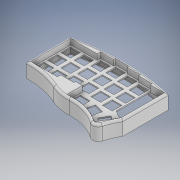
# Autodesk Inventor part: curvy
Saved by Autodesk Inventor 2021 (Build 250183000, 183)
## iProperties
Created: 2022-05-13
Part Number: curvy
Material: Generic
Document SubType Name: Modeling
Designer: Mark
Density: 1 g/cm^3
Appearance: Default
Author: Mark
Autodesk Inventor part; units mm, degrees
ref_plane "YZ Plane" through (0, 0, 0) normal (1, 0, 0) x (0, 1, 0)
ref_plane "XZ Plane" through (0, 0, 0) normal (0, 1, 0) x (-1, 0, 0)
ref_plane "XY Plane" through (0, 0, 0) normal (0, 0, 1) x (1, 0, 0)
sketch "keyholes" plane through (0, 0, 0) normal (0, 0, 1) x (1, 0, 0)
  line L0 (76.8681, -69.6062) -> (62.8681, -69.6062)
  line L1 (62.8681, -69.6062) -> (62.8681, -55.6062)
  line L2 (62.8681, -55.6062) -> (76.8681, -55.6062)
  line L3 (76.8681, -55.6062) -> (76.8681, -69.6062)
  line L4 (76.8681, -50.6062) -> (62.8681, -50.6062)
  line L5 (62.8681, -50.6062) -> (62.8681, -36.6062)
  line L6 (62.8681, -36.6062) -> (76.8681, -36.6062)
  line L7 (76.8681, -36.6062) -> (76.8681, -50.6062)
  line L8 (76.8681, -31.6062) -> (62.8681, -31.6062)
  line L9 (62.8681, -31.6062) -> (62.8681, -17.6062)
  line L10 (62.8681, -17.6062) -> (76.8681, -17.6062)
  line L11 (76.8681, -17.6062) -> (76.8681, -31.6062)
  point P0 (69.8681, -43.6062)
  dimension "d0" = 14
  dimension "d1" = 14
  dimension "d2" = 14
  dimension "d3" = 14
  dimension "d4" = 14
  dimension "d5" = 14
  dimension "d6" = 5
  dimension "d7" = 5
  measures "d0" distance of L1.end L2.end
  measures "d1" distance of L0.end L1.end
  measures "d2" distance of L5.end L6.end
  measures "d3" distance of L4.end L5.end
  measures "d4" distance of L9.end L10.end
  measures "d5" distance of L8.end L9.end
  measures "d6" distance between parallel lines of L4 L2
  measures "d7" distance between parallel lines of L8 L6
sketch "Sketch1" plane through (0, 0, 0) normal (0, 1, 0) x (-1, 0, 0)
  line L0 (119.155, -84.8943) -> (82.155, -84.8943) construction
  line L1 (64.1602, -28.6437) -> (119.155, -28.6437) construction
  line L2 (119.655, -29.1437) -> (119.655, -84.3943) construction
  line L3 (81.655, -85.3943) -> (81.655, -89.1443) construction
  line L4 (81.155, -89.6443) -> (63.155, -89.6443) construction
  line L5 (62.655, -90.1443) -> (62.655, -91.3943) construction
  line L6 (62.155, -91.8943) -> (45.155, -91.8943) construction
  line L7 (44.655, -91.3943) -> (44.655, -90.1443) construction
  line L8 (44.155, -89.6443) -> (26.155, -89.6443) construction
  line L9 (25.655, -89.1443) -> (25.655, -87.645) construction
  line L10 (25.155, -87.145) -> (7.155, -87.145) construction
  line L11 (63.7562, -28.4383) -> (53.3017, -14.1027) construction
  line L12 (52.9623, -13.9015) -> (15.7765, -9.0643) construction
  line L13 (15.591, -9.0015) -> (0.433, -0.25) construction
  line L14 (-0.25, -0.433) -> (-13.766, -23.8434) construction
  line L15 (-13.766, -23.8434) -> (6.655, -35.6335) construction
  line L16 (51.1256, -15.8625) -> (37.1256, -15.8625)
  line L17 (37.1256, -15.8625) -> (37.1256, -29.8625)
  line L18 (37.1256, -29.8625) -> (51.1256, -29.8625)
  line L19 (51.1256, -29.8625) -> (51.1256, -15.8625)
  line L20 (28.1127, -28.7255) -> (14.5898, -25.1021)
  line L21 (14.5898, -25.1021) -> (18.2132, -11.5791)
  line L22 (18.2132, -11.5791) -> (31.7362, -15.2026)
  line L23 (31.7362, -15.2026) -> (28.1127, -28.7255)
  line L24 (6.155, -84.895) -> (-13.5994, -84.895) construction
  line L25 (-14.0994, -84.395) -> (-14.0994, -24.5548) construction
  line L26 (-13.766, -23.8434) -> (-14.0324, -24.3048) construction
  line L27 (-8.6572, -18.9744) -> (-1.6572, -6.85)
  line L28 (3.4672, -25.9744) -> (-8.6572, -18.9744)
  line L29 (-1.6572, -6.85) -> (10.4672, -13.85)
  line L30 (10.4672, -13.85) -> (3.4672, -25.9744)
  arc A0 (119.155, -84.8943) -> (119.655, -84.3943) centre (119.155, -84.3943) ccw construction
  arc A1 (82.155, -84.8943) -> (81.655, -85.3943) centre (82.155, -85.3943) ccw construction
  arc A2 (81.155, -89.6443) -> (81.655, -89.1443) centre (81.155, -89.1443) ccw construction
  arc A3 (62.155, -91.8943) -> (62.655, -91.3943) centre (62.155, -91.3943) ccw construction
  arc A4 (44.655, -90.1443) -> (44.155, -89.6443) centre (44.155, -90.1443) ccw construction
  arc A5 (44.655, -91.3943) -> (45.155, -91.8943) centre (45.155, -91.3943) ccw construction
  arc A6 (63.155, -89.6443) -> (62.655, -90.1443) centre (63.155, -90.1443) ccw construction
  arc A7 (25.655, -89.1443) -> (26.155, -89.6443) centre (26.155, -89.1443) ccw construction
  arc A8 (-14.0994, -84.395) -> (-13.5994, -84.895) centre (-13.5994, -84.395) ccw construction
  line L31 (6.655, -86.645) -> (6.655, -85.395) construction
  arc A9 (25.655, -87.645) -> (25.155, -87.145) centre (25.155, -87.645) ccw construction
  arc A10 (6.655, -86.645) -> (7.155, -87.145) centre (7.155, -86.645) ccw construction
  arc A11 (6.655, -85.395) -> (6.155, -84.895) centre (6.155, -85.395) ccw construction
  arc A12 (-14.0324, -24.3048) -> (-14.0994, -24.5548) centre (-13.5994, -24.5548) ccw construction
  arc A13 (0.433, -0.25) -> (-0.25, -0.433) centre (0.183, -0.683) ccw construction
  arc A14 (15.591, -9.0015) -> (15.7765, -9.0643) centre (15.841, -8.5685) ccw construction
  arc A15 (53.3017, -14.1027) -> (52.9623, -13.9015) centre (52.8978, -14.3973) ccw construction
  arc A16 (63.7562, -28.4383) -> (64.1602, -28.6437) centre (64.1602, -28.1437) ccw construction
  arc A17 (119.655, -29.1437) -> (119.155, -28.6437) centre (119.155, -29.1437) ccw construction
  line L32 (6.655, -35.6335) -> (6.655, -85.395) construction
  line L33 (120.144, -28.2713) -> (120.144, -85.2713)
  line L34 (120.144, -85.2713) -> (82.144, -85.2713)
  line L35 (82.144, -85.2713) -> (82.144, -90.0161)
  line L36 (82.144, -90.0161) -> (63.144, -90.0161)
  line L37 (63.144, -90.0161) -> (63.144, -92.395)
  line L38 (63.144, -92.395) -> (44.144, -92.395)
  line L39 (44.144, -92.395) -> (44.144, -90.0204)
  line L40 (44.144, -90.0204) -> (25.144, -90.0204)
  line L41 (25.144, -90.0204) -> (25.144, -87.6356)
  line L42 (25.144, -87.6356) -> (6.144, -87.6356)
  line L43 (120.144, -28.2713) -> (82.144, -28.2713)
  line L44 (82.144, -28.2713) -> (82.144, -33.0161)
  line L45 (82.144, -33.0161) -> (63.144, -33.0161)
  line L46 (63.144, -33.0161) -> (63.144, -35.395)
  line L47 (63.144, -35.395) -> (53.6256, -35.395)
  line L48 (53.6256, -35.395) -> (53.6256, -13.3625)
  line L49 (53.6256, -13.3625) -> (34.5282, -13.3625)
  line L50 (34.5282, -13.3625) -> (16.0445, -8.4098)
  line L51 (16.0445, -8.4098) -> (-0.0722, 0.8952)
  line L52 (-0.0722, 0.8952) -> (-14.5722, -24.2195)
  line L53 (-14.5722, -24.2195) -> (6.144, -36.1801)
  line L54 (6.144, -36.1801) -> (6.144, -87.6356)
  line L55 (6.155, -84.895) -> (-14.0994, -84.895)
  arc A18 (73.017, -18.1715) -> (120.144, -28.2713) centre (120.144, 86.7287) ccw
  arc A19 (-14.0994, -84.895) -> (120.144, -85.2713) centre (53.8578, 212.9425) ccw
  arc A20 (-0.0722, 0.8952) -> (53.6256, -13.3625) centre (44.1644, 59.2526) ccw construction
  arc A21 (2.09, 0.0448) -> (47.4821, -13.3064) centre (44.1644, 59.2526) ccw
  arc A22 (-14.0994, -23.4005) -> (-5.3538, -2.5918) centre (-92.0416, 21.5995) ccw
  line L56 (-14.0994, -84.895) -> (-14.0994, -23.4005)
  arc A23 (73.017, -18.1715) -> (47.4821, -13.3064) centre (50.0429, -69.3097) ccw
  arc A24 (2.09, 0.0448) -> (-5.3538, -2.5918) centre (-0.7055, -3.889) ccw
  line L57 (98.644, -82.7713) -> (84.644, -82.7713)
  line L58 (84.644, -82.7713) -> (84.644, -68.7713)
  line L59 (84.644, -68.7713) -> (98.644, -68.7713)
  line L60 (98.644, -68.7713) -> (98.644, -82.7713)
  line L61 (98.644, -63.7713) -> (84.644, -63.7713)
  line L62 (84.644, -63.7713) -> (84.644, -49.7713)
  line L63 (84.644, -49.7713) -> (98.644, -49.7713)
  line L64 (98.644, -49.7713) -> (98.644, -63.7713)
  line L65 (98.644, -44.7713) -> (84.644, -44.7713)
  line L66 (84.644, -44.7713) -> (84.644, -30.7713)
  line L67 (84.644, -30.7713) -> (98.644, -30.7713)
  line L68 (98.644, -30.7713) -> (98.644, -44.7713)
  line L69 (117.644, -82.7713) -> (103.644, -82.7713)
  line L70 (103.644, -82.7713) -> (103.644, -68.7713)
  line L71 (103.644, -68.7713) -> (117.644, -68.7713)
  line L72 (117.644, -68.7713) -> (117.644, -82.7713)
  line L73 (117.644, -63.7713) -> (103.644, -63.7713)
  line L74 (103.644, -63.7713) -> (103.644, -49.7713)
  line L75 (103.644, -49.7713) -> (117.644, -49.7713)
  line L76 (117.644, -49.7713) -> (117.644, -63.7713)
  line L77 (117.644, -44.7713) -> (103.644, -44.7713)
  line L78 (103.644, -44.7713) -> (103.644, -30.7713)
  line L79 (103.644, -30.7713) -> (117.644, -30.7713)
  line L80 (117.644, -30.7713) -> (117.644, -44.7713)
  line L81 (79.644, -87.5161) -> (65.644, -87.5161)
  line L82 (65.644, -87.5161) -> (65.644, -73.5161)
  line L83 (65.644, -73.5161) -> (79.644, -73.5161)
  line L84 (79.644, -73.5161) -> (79.644, -87.5161)
  line L85 (79.644, -68.5161) -> (65.644, -68.5161)
  line L86 (65.644, -68.5161) -> (65.644, -54.5161)
  line L87 (65.644, -54.5161) -> (79.644, -54.5161)
  line L88 (79.644, -54.5161) -> (79.644, -68.5161)
  line L89 (79.644, -49.5161) -> (65.644, -49.5161)
  line L90 (65.644, -49.5161) -> (65.644, -35.5161)
  line L91 (65.644, -35.5161) -> (79.644, -35.5161)
  line L92 (79.644, -35.5161) -> (79.644, -49.5161)
  line L93 (60.644, -89.895) -> (46.644, -89.895)
  line L94 (46.644, -89.895) -> (46.644, -75.895)
  line L95 (46.644, -75.895) -> (60.644, -75.895)
  line L96 (60.644, -75.895) -> (60.644, -89.895)
  line L97 (60.644, -70.895) -> (46.644, -70.895)
  line L98 (46.644, -70.895) -> (46.644, -56.895)
  line L99 (46.644, -56.895) -> (60.644, -56.895)
  line L100 (60.644, -56.895) -> (60.644, -70.895)
  line L101 (60.644, -51.895) -> (46.644, -51.895)
  line L102 (46.644, -51.895) -> (46.644, -37.895)
  line L103 (46.644, -37.895) -> (60.644, -37.895)
  line L104 (60.644, -37.895) -> (60.644, -51.895)
  line L105 (41.644, -87.5204) -> (27.644, -87.5204)
  line L106 (27.644, -87.5204) -> (27.644, -73.5204)
  line L107 (27.644, -73.5204) -> (41.644, -73.5204)
  line L108 (41.644, -73.5204) -> (41.644, -87.5204)
  line L109 (41.644, -68.5204) -> (27.644, -68.5204)
  line L110 (27.644, -68.5204) -> (27.644, -54.5204)
  line L111 (27.644, -54.5204) -> (41.644, -54.5204)
  line L112 (41.644, -54.5204) -> (41.644, -68.5204)
  line L113 (41.644, -49.5204) -> (27.644, -49.5204)
  line L114 (27.644, -49.5204) -> (27.644, -35.5204)
  line L115 (27.644, -35.5204) -> (41.644, -35.5204)
  line L116 (41.644, -35.5204) -> (41.644, -49.5204)
  line L117 (22.644, -85.1356) -> (8.644, -85.1356)
  line L118 (8.644, -85.1356) -> (8.644, -71.1356)
  line L119 (8.644, -71.1356) -> (22.644, -71.1356)
  line L120 (22.644, -71.1356) -> (22.644, -85.1356)
  line L121 (22.644, -66.1356) -> (8.644, -66.1356)
  line L122 (8.644, -66.1356) -> (8.644, -52.1356)
  line L123 (8.644, -52.1356) -> (22.644, -52.1356)
  line L124 (22.644, -52.1356) -> (22.644, -66.1356)
  line L125 (22.644, -47.1356) -> (8.644, -47.1356)
  line L126 (8.644, -47.1356) -> (8.644, -33.1356)
  line L127 (8.644, -33.1356) -> (22.644, -33.1356)
  line L128 (22.644, -33.1356) -> (22.644, -47.1356)
  point P0 (119.655, -84.8943)
  point P1 (63.906, -28.6437)
  point P2 (81.655, -84.8943)
  point P3 (119.655, -28.6437)
  point P4 (81.655, -89.6443)
  point P5 (62.655, -89.6443)
  point P6 (62.655, -91.8943)
  point P7 (44.655, -91.8943)
  point P8 (44.655, -89.6443)
  point P9 (25.655, -89.6443)
  point P10 (25.655, -87.145)
  point P11 (53.1752, -13.9292)
  point P12 (15.6775, -9.0514)
  point P13 (0, 0)
  point P14 (0, 0)
  point P15 (6.655, -87.145)
  point P16 (0, 0)
  point P17 (6.144, -84.895)
  point P18 (45.8572, -13.3625)
  point P19 (25.3651, -10.9073)
  point P20 (42.4716, -13.3625)
  point P21 (-14.0994, -24.4926)
  dimension "d8" = 5
  dimension "d14" = 4.7448
  dimension "d15" = 5
  dimension "d18" = 2.3788
  dimension "d19" = 5
  dimension "d22" = 5
  dimension "d23" = 5
  dimension "d24" = 2.3746
  dimension "d25" = 2.3849
  dimension "d9" = 2.123
  dimension "d10" = 2.011
  dimension "d11" = 38
  dimension "d12" = 4.75
  dimension "d13" = 2.1277
  dimension "d16" = 19
  dimension "d17" = 2.25
  dimension "d20" = 18
  dimension "d21" = 2.25
  dimension "d26" = 19
  dimension "d27" = 19
  dimension "d28" = 55.749
  dimension "d29" = 18.2117
  dimension "d30" = 126.102
  dimension "d31" = 133.514
  dimension "d32" = 37.8137
  dimension "d33" = 18.1028
  dimension "d34" = 27.532
  dimension "d35" = 14
  dimension "d36" = 14
  dimension "d37" = 5.6579
  dimension "d38" = 4.5184
  dimension "d39" = 14
  dimension "d40" = 14
  dimension "d41" = 15
  dimension "d42" = 5.3894
  dimension "d43" = 1.137
  dimension "d44" = 2.25
  dimension "d45" = 14
  dimension "d46" = 14
  dimension "d47" = 30
  dimension "d48" = 7.7461
  dimension "d49" = 11.2521
  dimension "d50" = 90
  dimension "d51" = 90
  dimension "d52" = 2.4994
  dimension "d53" = 0.5
  dimension "d54" = 0.5
  dimension "d55" = 0.5
  dimension "d56" = 0.5
  dimension "d57" = 20.7543
  dimension "d61" = 2.5
  dimension "d62" = 2.5
  dimension "d63" = 2.5
  dimension "d64" = 2.5
  dimension "d65" = 2.5
  dimension "d66" = 2.5
  dimension "d67" = 2.5
  dimension "d68" = 2.5
  dimension "d69" = 2.5
  dimension "d70" = 2.5
  dimension "d71" = 2.5
  dimension "d72" = 2.5
  dimension "d73" = 2.5
  dimension "d74" = 2.5
  dimension "d75" = 2.5
  dimension "d76" = 2.5
  dimension "d77" = 2.5
  dimension "d78" = 2.5
  dimension "d79" = 2.5
  dimension "d80" = 2.5
  dimension "d81" = 7.5
  dimension "d82" = 7.5
  dimension "d85" = 73.2289
  constraints: 112 end point, 54 point on circle, 43 tangent, 34 point on line, 25 centre point, 24 perpendicular, 14 equal radius, 12 parallel, 7 horizontal, 5 vertical, 3 coincident, 1 collinear, 3 other
  measures "d11" distance of point (119.655, -84.894) point (81.655, -84.894)
  measures "d12" distance of point (81.655, -84.894) point (81.655, -89.644)
  measures "d16" distance of point (81.655, -89.644) point (62.655, -89.644)
  measures "d17" distance between parallel lines of L6 L4
  measures "d20" distance of point (62.655, -91.894) point (44.655, -91.894)
  measures "d21" distance of point (44.655, -91.894) point (44.655, -89.644)
  measures "d26" distance of point (44.655, -89.644) point (25.655, -89.644)
  measures "d27" distance of point (6.655, -87.145) point (25.655, -87.145)
  measures "d28" distance of point (63.906, -28.644) point (119.655, -28.644)
  measures "d29" distance of point (63.906, -28.644) point (53.175, -13.929)
  measures "d30" angle of L11 L1
  measures "d31" angle of L12 L11
  measures "d32" distance of point (53.175, -13.929) point (15.677, -9.051)
  measures "d33" distance of point (15.677, -9.051) point (0, 0)
  measures "d34" distance of point (0, 0) L26.start
  measures "d35" distance of L19.start L17.end
  measures "d36" distance of L17.end L17.start
  measures "d39" distance of L22.start L23.start
  measures "d40" distance of L20.end L22.start
  measures "d41" angle of L23 L17
  measures "d42" horizontal distance of L23.start L17.start
  measures "d43" vertical distance of L23.end L17.end
  measures "d44" distance between parallel lines of L24 L10
  measures "d45" distance of L29.start L30.start
  measures "d46" distance of L27.start L29.start
  measures "d47" angle of L17 L30
  measures "d48" horizontal distance of L30.start L22.start
  measures "d49" vertical distance of L30.start L20.end
  measures "d50" angle of L14 L13
  measures "d52" distance of point (25.655, -89.644) point (25.655, -87.145)
  measures "d53" radius of A0
  measures "d54" radius of A3
  measures "d55" radius of A9
  measures "d56" radius of A8
  measures "d57" distance between parallel lines of L25 L31
  measures "d73" distance between parallel lines of L22 L50
  measures "d74" distance between parallel lines of L16 L49
  measures "d75" distance between parallel lines of L48 L19
  measures "d80" distance between parallel lines of L52 L27
  measures "d81" distance between parallel lines of L51 L29
  measures "d82" distance between parallel lines of L53 L28
  measures "d85" radius of A20
sketch "Sketch2" plane through (0, 0, 0) normal (0, 1, 0) x (-1, 0, 0)
  arc A0 (-14.0994, -84.895) -> (120.144, -85.2713) centre (53.8578, 212.9425) ccw projected
  line L0 (120.144, -28.2713) -> (120.144, -85.2713) projected
  arc A1 (73.017, -18.1715) -> (120.144, -28.2713) centre (120.144, 86.7287) ccw projected
  arc A2 (73.017, -18.1715) -> (47.4821, -13.3064) centre (50.0429, -69.3097) ccw projected
  arc A3 (2.09, 0.0448) -> (47.4821, -13.3064) centre (44.1644, 59.2526) ccw projected
  arc A4 (2.09, 0.0448) -> (-5.3538, -2.5918) centre (-0.7055, -3.889) ccw projected
  arc A5 (-14.0994, -23.4005) -> (-5.3538, -2.5918) centre (-92.0416, 21.5995) ccw projected
  line L1 (-14.0994, -84.895) -> (-14.0994, -23.4005) projected
  arc A6 (-17.0994, -87.278) -> (123.144, -87.6681) centre (53.8578, 212.9425) ccw
  line L2 (-17.0994, -87.278) -> (-17.0994, -22.5893)
  arc A7 (-17.0994, -22.5893) -> (-8.2434, -1.7855) centre (-92.0416, 21.5995) ccw
  arc A8 (3.8277, 2.4902) -> (-8.2434, -1.7855) centre (-0.7055, -3.889) ccw
  arc A9 (3.8277, 2.4902) -> (47.3451, -10.3096) centre (44.1644, 59.2526) ccw
  arc A10 (74.2464, -15.435) -> (47.3451, -10.3096) centre (50.0429, -69.3097) ccw
  arc A11 (74.2464, -15.435) -> (123.144, -25.2311) centre (120.144, 86.7287) ccw
  line L3 (123.144, -25.2311) -> (123.144, -87.6681)
  point P0 (0, 0)
  dimension "d89" = 3
  constraints: 12 point on circle, 6 centre point, 4 end point, 7 other
  measures "d89" radial gap between concentric circles of A0 A6
extrude "Extrusion1" add sketch "Sketch1" along normal blind 9.5 contours L43 L44 L45 L46 L47 L48 A23 A18 | A19 L38 L37 L36 L35 L34 | A19 L55 L54 L42 L41 L40 L39 | L49 A21 A23 | L49 L50 A21 | A22 A24 L52 | L50 L51 A24 A21
extrude "Extrusion2" add sketch "Sketch2" along normal blind 9.5
extrude "Extrusion3" add sketch "Sketch1" along normal blind 1.5 contours L33 L34 L35 L36 L37 L38 L39 L40 L41 L42 L54 L53 L56 L52 L51 L50 L49 A21 L48 L47 L46 L45 L44 L43
extrude "Extrusion4" add sketch "Sketch2" against normal blind 11.5
fillet "Fillet1" radius 3 8 edges at (-61.0969, 9.5, -11.2916) (-24.515, 9.5, -7.5524) (3.3184, 9.5, 3.4878) (11.9927, 9.5, -12.4763) (-98.143, 9.5, -23.0892) (17.0994, 9.5, -54.9337) (-52.9999, 9.5, -95.5483) (-123.144, 9.5, -56.4496)
sketch "Sketch3" plane through (0, -11.5, 0) normal (0, -1, 0) x (1, 0, 0)
  arc A0 (-123.144, -87.6681) -> (17.0994, -87.278) centre (-53.8578, 212.9425) ccw projected
  line L0 (17.0994, -87.278) -> (17.0994, -22.5893) projected
  arc A1 (8.2434, -1.7855) -> (17.0994, -22.5893) centre (92.0416, 21.5995) ccw projected
  arc A2 (8.2434, -1.7855) -> (-3.8277, 2.4902) centre (0.7055, -3.889) ccw projected
  arc A3 (-47.3451, -10.3096) -> (-3.8277, 2.4902) centre (-44.1644, 59.2526) ccw projected
  arc A4 (-47.3451, -10.3096) -> (-74.2464, -15.435) centre (-50.0429, -69.3097) ccw projected
  arc A5 (-123.144, -25.2311) -> (-74.2464, -15.435) centre (-120.144, 86.7287) ccw projected
  line L1 (-123.144, -25.2311) -> (-123.144, -87.6681) projected
  arc A6 (5.3538, -2.5918) -> (14.0994, -23.4005) centre (92.0416, 21.5995) ccw projected
  line L2 (14.0994, -23.4005) -> (14.0994, -84.895) projected
  arc A7 (-120.144, -85.2713) -> (14.0994, -84.895) centre (-53.8578, 212.9425) ccw projected
  line L3 (-120.144, -85.2713) -> (-120.144, -28.2713) projected
  arc A8 (-120.144, -28.2713) -> (-73.017, -18.1715) centre (-120.144, 86.7287) ccw projected
  arc A9 (-47.4821, -13.3064) -> (-73.017, -18.1715) centre (-50.0429, -69.3097) ccw projected
  arc A10 (-47.4821, -13.3064) -> (-2.09, 0.0448) centre (-44.1644, 59.2526) ccw projected
  arc A11 (5.3538, -2.5918) -> (-2.09, 0.0448) centre (0.7055, -3.889) ccw projected
  arc A12 (-121.644, -26.7614) -> (-73.6317, -16.8032) centre (-120.144, 86.7287) ccw
  line L4 (-121.644, -26.7614) -> (-121.644, -86.4721)
  arc A13 (-121.644, -86.4721) -> (15.5994, -86.0889) centre (-53.8578, 212.9425) ccw
  line L5 (15.5994, -86.0889) -> (15.5994, -22.9967)
  arc A14 (6.7986, -2.1887) -> (15.5994, -22.9967) centre (92.0416, 21.5995) ccw
  arc A15 (6.7986, -2.1887) -> (-2.9589, 1.2675) centre (0.7055, -3.889) ccw
  arc A16 (-47.4136, -11.808) -> (-2.9589, 1.2675) centre (-44.1644, 59.2526) ccw
  arc A17 (-47.4136, -11.808) -> (-73.6317, -16.8032) centre (-50.0429, -69.3097) ccw
  point P0 (0, 0)
  dimension "d99" = 1.5
  constraints: 12 point on circle, 6 centre point, 4 end point, 7 other
  measures "d99" radial gap between concentric circles of A9 A17
extrude "Extrusion5" cut sketch "Sketch3" against normal blind 3 contours A12 A17 A16 A15 A14 L5 A13 L4
body "Solid1"
